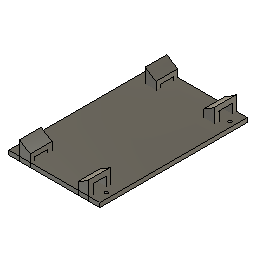
Adaptador PCB-ROBOT (Autodesk Fusion 360 design; units mm, degrees)
part number: 2025-12-06-18-00-58-751
Autodesk Fusion 360 part; units mm, degrees
note: some values were not read from the file. Set by a fixed rule: which face or edge a step refers to.
sketch "Boceto1" plane through (0, 0, 0) normal (0, 0, 1) x (1, 0, 0)
sketch "Boceto2" plane through (0, 0, 0) normal (0, 0, 1) x (1, 0, 0)
  line L0 (0, 0) -> (80, 0)
  line L1 (80, 0) -> (80, 120)
  line L2 (80, 120) -> (0, 120)
  line L3 (0, 120) -> (0, 0)
  dimension "d1" = 120
  dimension "d2" = 80
  constraint horizontal L0
  constraint vertical L1
  constraint horizontal L2
  constraint vertical L3
  constraint coincident L0.start L3.end
  measures "d1" distance of L0.end L1.end
  measures "d2" distance of L1.end L2.end
sketch "Boceto3" plane through (0, 0, 0) normal (0, 1, 0) x (1, 0, 0)
sketch "Boceto4" plane through (0, 0, 6) normal (0, 0, 1) x (-1, 0, 0)
  line L0 (0, -120) -> (0, 0)
  line L1 (0, 0) -> (-80, 0)
  line L2 (-80, 0) -> (-80, -120)
  line L3 (-80, -120) -> (0, -120)
sketch "Boceto5" plane through (0, 0, 0) normal (1, 0, 0) x (0, 1, 0)
sketch "Boceto6" plane through (0, 0, 6) normal (0, 0, 1) x (-1, 0, 0)
sketch "Boceto7" plane through (0, 0, 0) normal (0, 0, 1) x (1, 0, 0)
sketch "Boceto8" plane through (0, 0, 0) normal (0, 0, 1) x (1, 0, 0)
sketch "Boceto9" plane through (0, 0, 0) normal (0, 0, 1) x (1, 0, 0)
  line L0 (75, -55) -> (70, -55)
  line L1 (70, -55) -> (70, -40)
  line L2 (70, -40) -> (75, -40)
  line L3 (75, -40) -> (75, -55)
  dimension "d5" = 15
  constraint horizontal L0
  constraint vertical L1
  constraint horizontal L2
  constraint vertical L3
  measures "d5" distance of L0.start L2.end
sketch "Boceto10" plane through (0, 0, 0) normal (0, 0, 1) x (1, 0, 0)
  line L0 (-60, -66) -> (-60, -40)
  line L1 (-60, -40) -> (-50, -40)
  line L2 (-50, -40) -> (-50, -56.8)
  spline S0 degree 5 poles (-50, -56.8) (-50.2369, -56.8317) (-50.7073, -56.9088) (-51.4028, -57.0651) (-52.3097, -57.3562) (-53.4068, -57.8667) (-54.4648, -58.535) (-55.4814, -59.3704) (-56.4566, -60.3722) (-57.3935, -61.5284) (-58.2956, -62.8249) (-58.9921, -63.9639) (-59.5011, -64.8716) (-59.8347, -65.5001) (-60, -65.8202) knots 0 0 0 0 0 0 0.1 0.2 0.3 0.4 0.5 0.6 0.7 0.8 0.9 1 1 1 1 1 1
  line L3 (-60, -66) -> (-60, -65.8202)
  point P0 (-55, -59)
  dimension "d8" = 26
  dimension "d9" = 16.8
  dimension "d10" = 10
  constraint vertical L0
  constraint perpendicular L0 L1
  constraint perpendicular L1 L2
  measures "d8" distance of L0.start L0.end
  measures "d9" distance of L1.end L2.end
  measures "d10" distance of L0.end L1.end
sketch "Boceto11" plane through (0, 0, 0) normal (0, 0, -1) x (1, 0, 0)
  line L0 (80, -120) -> (80, 0)
  line L1 (0, 8) -> (80, 8)
  line L2 (80, -128) -> (0, -128)
  line L3 (40, -128) -> (40, 8) construction
  line L4 (0, -60) -> (80, -60) construction
  circle A0 centre (77, -3) radius 1.5
  circle A1 centre (3, -3) radius 1.5
  circle A2 centre (77, -117) radius 1.5
  circle A3 centre (3, -117) radius 1.5
  line L5 (0, -128) -> (-2, -128)
  line L6 (0, 8) -> (-2, 8)
  line L7 (-2, 8) -> (-2, -128)
  line L8 (80, -128) -> (82, -128)
  line L9 (82, -128) -> (82, 8)
  line L10 (82, 8) -> (80, 8)
  point P0 (77, -117)
  point P1 (3, -117)
  dimension "d172" = 136
  dimension "d173" = 136
  dimension "d174" = 80
  dimension "d175" = 80
  dimension "d210" = 3
  constraint midpoint L2 L3.start
  constraint midpoint L1 L3.end
  constraint perpendicular L1 L3
  constraint symmetric L3 A0 A1
  constraint symmetric L4 A0.centre P0
  constraint symmetric L4 A1.centre P1
  constraint coincident P0 A2.centre
  constraint coincident P1 A3.centre
  constraint perpendicular L5 L7
  constraint perpendicular L8 L9
  measures "d172" distance of L2.end L1.start
  measures "d173" distance of L1.end L2.start
  measures "d174" distance of L2.end L2.start
  measures "d175" distance of L1.start L1.end
  measures "d210" diameter of A0
sketch "Boceto12" plane through (0, 0, 0) normal (0, 0, 1) x (1, 0, 0)
sketch "Boceto13" plane through (0, 0, 0) normal (0, 0, 1) x (1, 0, 0)
  line L0 (0, 0) -> (30, 0)
  spline S0 degree 5 poles (40, 31.6386) (39.8106, 31.8697) (39.4308, 32.3285) (38.8584, 33.0066) (38.0897, 33.8902) (37.1188, 34.9583) (36.1372, 35.9864) (35.1438, 36.9711) (34.1379, 37.9101) (33.12, 38.8045) (32.0909, 39.6576) (31.2594, 40.3096) (30.6314, 40.7826) (30.2108, 41.0908) (30, 41.2432) knots 0 0 0 0 0 0 0.1 0.2 0.3 0.4 0.5 0.6 0.7 0.8 0.9 1 1 1 1 1 1
  line L1 (40, 31.6386) -> (40, 57.6386)
  line L2 (40, 57.6386) -> (30, 57.6386)
  line L3 (30, 57.6386) -> (30, 41.2432)
  point P0 (35.0003, 37.0942)
  dimension "d178" = 26
  dimension "d179" = 10
  dimension "d180" = 16.3954
  constraint coincident L0.start origin
  constraint horizontal L0
  constraint vertical L1
  constraint perpendicular L1 L2
  constraint perpendicular L2 L3
  measures "d178" distance of S0.start L1.end
  measures "d179" distance of L1.end L2.end
  measures "d180" distance of S0.end L2.end
sketch "Boceto14" plane through (0, 0, 0) normal (0, 1, 0) x (1, 0, 0)
sketch "Boceto15" plane through (0, 0, 0) normal (0, 1, 0) x (1, 0, 0)
sketch "Boceto16" plane through (0, 0, 0) normal (0, 1, 0) x (1, 0, 0)
sketch "Boceto17" plane through (0, 0, 0) normal (0, 1, 0) x (1, 0, 0)
  circle A0 centre (40, -52) radius 51
extrude "Extruir19" add sketch "Boceto17" along normal blind 20 makes body 1
extrude "Extruir20" add sketch "Boceto11" along normal blind 4 separate body makes body 2
move_body "Desplazar87" bodies 2 to x (1, 0, 0) y (0, 1, 0) z (0, 0, 1) at (0, 150, 0)
move_body "Desplazar88" bodies 1 to x (1, 0, 0) y (0, 1, 0) z (0, 0, 1) at (-40, 0, 0)
move_body "Desplazar89" bodies 2 to x (1, 0, 0) y (0, 1, 0) z (0, 0, 1) at (-40, 0, 0)
move_body "Desplazar90" bodies 2 to x (1, 0, 0) y (0, 1, 0) z (0, 0, 1) at (0, 0, 50)
move_body "Desplazar91" bodies 2 to x (1, 0, 0) y (0, 1, 0) z (0, 0, 1) at (0, 0, -50)
sketch "Boceto18" plane through (0, 20, 0) normal (0, 1, 0) x (-1, 0, 0)
  circle A0 centre (0, 52) radius 51
  spline S0 degree 5 poles (-32.01, 12.2966) (-31.8149, 12.1431) (-31.4244, 11.8383) (-30.8372, 11.3883) (-30.0516, 10.8029) (-29.0648, 10.0969) (-28.0728, 9.419) (-27.0752, 8.7718) (-26.0716, 8.1567) (-25.0624, 7.5726) (-24.0478, 7.0173) (-23.2322, 6.5943) (-22.6184, 6.2882) (-22.2084, 6.089) (-22.0031, 5.9906) knots 0 0 0 0 0 0 0.1 0.2 0.3 0.4 0.5 0.6 0.7 0.8 0.9 1 1 1 1 1 1
  line L0 (-32.01, 12.2966) -> (-32.01, 0)
  line L1 (-32.01, 0) -> (-22, 0)
  line L2 (-22, 0) -> (-22.0031, 5.9906)
  point P0 (-26.9896, 8.7269)
  constraint coincident A0 P0
  constraint coincident A0 S0.end
  constraint vertical L0
  constraint perpendicular L0 L1
move_body "Desplazar98" bodies 1 to x (1, 0, 0) y (0, 1, 0) z (0, 0, 1) at (0, 0, 5)
move_body "Desplazar103" bodies 1 to x (1, 0, 0) y (0, 1, 0) z (0, 0, 1) at (0, -4, 0)
move_body "Desplazar104" bodies 1 to x (1, 0, 0) y (0, 1, 0) z (0, 0, 1) at (0, 0, -4)
move_body "Desplazar109" bodies 1 to x (1, 0, 0) y (0, 1, 0) z (0, 0, 1) at (0, 0, 2)
extrude "Extruir33" add 1 faces at (16.2447, -4, 49.9892) along direction (0, -1, 0) blind 225 on bodies 1 bodies 1
move_body "Desplazar110" bodies 1 to x (1, 0, 0) y (0, 1, 0) z (0, 0, 1) at (0, 300, 0)
extrude "Extruir34" cut 1 faces at (16.2447, 316, 49.9892) along direction (0, -1, 0) blind 50 on bodies 1 bodies 1
move_body "Desplazar111" bodies 1 to x (1, 0, 0) y (0, 1, 0) z (0, 0, 1) at (0, 50, 0)
sketch "Boceto19" plane through (0, 316, 0) normal (0, 1, 0) x (-1, 0, 0)
  circle A0 centre (0, 55) radius 51
sketch "Boceto20" plane through (0, 316, 0) normal (0, 1, 0) x (-1, 0, 0)
  spline S0 degree 5 poles (-32, 15.3) (-31.8059, 15.1468) (-31.4171, 14.8426) (-30.8324, 14.3935) (-30.0497, 13.8091) (-29.0658, 13.1043) (-28.0759, 12.4274) (-27.0794, 11.781) (-26.0761, 11.1664) (-25.0662, 10.5826) (-24.0501, 10.0273) (-23.2327, 9.6041) (-22.6173, 9.2978) (-22.2059, 9.0985) (-22, 9) knots 0 0 0 0 0 0 0.1 0.2 0.3 0.4 0.5 0.6 0.7 0.8 0.9 1 1 1 1 1 1
  line L0 (-32, 15.3) -> (-32, -25)
  line L1 (-32, -25) -> (-22, -25)
  line L2 (-22, -25) -> (-22, 9)
  point P0 (-27, 11.74)
  constraint vertical L0
  constraint perpendicular L0 L1
extrude "Extruir35" add sketch "Boceto20" along normal blind 20 separate body makes body 3
shell "Vaciado9" thickness 4 removed faces 2 at (22, 322.6667, -13.6667) at (32, 329.3333, 1.8667) on bodies 3
move_body "Desplazar112" bodies 3 to x (1, 0, 0) y (0, 1, 0) z (0, 0, 1) at (0, -60, 0)
copy_body "CopiarPegarCuerpos14" bodies 3 makes body 4
move_body "Desplazar113" bodies 4 to x (1, 0, 0) y (0, 1, 0) z (0, 0, 1) at (0, 0, 0)
move_body "Desplazar114" bodies 4 to x (1, 0, 0) y (0, 1, 0) z (0, 0, 1) at (0, -115, 0)
move_body "Desplazar115" bodies 4 to x (1, 0, 0) y (0, 1, 0) z (0, 0, 1) at (0, 3, 0)
copy_body "CopiarPegarCuerpos15" bodies 4 makes body 5
move_body "Desplazar116" bodies 5 to x (1, 0, 0) y (0, 1, 0) z (0, 0, 1) at (0, 0, 0)
move_body "Desplazar117" bodies 5 to x (-1, 0, 0) y (0, -1, 0) z (0, 0, 1) at (-11.0179, 308, 0)
move_body "Desplazar119" bodies 5 to x (1, 0, 0) y (0, 1, 0) z (0, 0, 1) at (0, 112, 0)
copy_body "CopiarPegarCuerpos17" bodies 5 makes body 6
move_body "Desplazar120" bodies 6 to x (1, 0, 0) y (0, 1, 0) z (0, 0, 1) at (0, 0, 0)
move_body "Desplazar121" bodies 6 to x (1, 0, 0) y (0, 1, 0) z (0, 0, 1) at (0, -110, 0)
move_body "Desplazar122" bodies 6 5 to x (1, 0, 0) y (0, 1, 0) z (0, 0, 1) at (11, 0, 0)
move_body "Desplazar123" bodies 1 to x (1, 0, 0) y (0, 1, 0) z (0, 0, 1) at (0, 0, -3)
move_body "Desplazar124" bodies 5 6 to x (1, 0, 0) y (0, 1, 0) z (0, 0, 1) at (0, 0, -3)
move_body "Desplazar125" bodies 4 3 to x (1, 0, 0) y (0, 1, 0) z (0, 0, 1) at (0, 0, -3)
move_body "Desplazar126" bodies 4 6 5 3 1 to x (1, 0, 0) y (0, 1, 0) z (0, 0, 1) at (0, 0, 1)
move_body "Desplazar127" bodies 1 to x (1, 0, 0) y (0, 1, 0) z (0, 0, 1) at (0, 0, 100)
move_body "Desplazar128" bodies 3 to x (1, 0, 0) y (0, 1, 0) z (0, 0, 1) at (0, 2, 0)
move_body "Desplazar129" bodies 5 to x (1, 0, 0) y (0, 1, 0) z (0, 0, 1) at (0, 2, 0)
move_body "Desplazar130" bodies 4 to x (1, 0, 0) y (0, 1, 0) z (0, 0, 1) at (0, -2, 0)
move_body "Desplazar131" bodies 6 to x (1, 0, 0) y (0, 1, 0) z (0, 0, 1) at (0, -4, 0)
move_body "Desplazar132" bodies 1 to x (1, 0, 0) y (0, 1, 0) z (0, 0, 1) at (0, 0, -100)
extrude "Extruir36" cut 1 faces at (-28.6845, 155.3333, -27) along direction (0, 0, 1) blind 23 on bodies 6 bodies 6
extrude "Extruir37" cut 1 faces at (28.6667, 148.6667, -27) along direction (0, 0, 1) blind 23 on bodies 4 bodies 4
extrude "Extruir38" cut 1 faces at (28.6667, 264.6667, -27) along direction (0, 0, 1) blind 23 on bodies 3 bodies 3
extrude "Extruir39" cut 1 faces at (-28.6845, 271.3333, -27) along direction (0, 0, 1) blind 23 on bodies 5 bodies 5
hidden bodies 1
named bodies: "Brazo-Robot", "Base", "Patilla 1", "Patilla 2", "Patilla 3", "Patilla 4"
